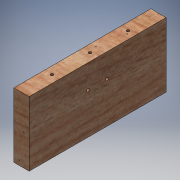
# Autodesk Inventor part: licht_200_side_left
Saved by Autodesk Inventor 2016 SP2 (Build 200236200, 236)
## iProperties
Created: 2018-01-11
Part Number: licht_200_side_left
Material: Spanplatte
Document SubType Name: Blech
Designer: schueler
Density: 1 g/cm^3
Sheet Metal Rule: Standard_mm
Appearance: Birke - natur- poliert
Mass: 154.711 g
Surface Area: 288.071 cm^2
Volume: 154.711 cm^3
Author: schueler
Autodesk Inventor part; units mm, degrees
ref_plane "YZ Plane" through (0, 0, 0) normal (1, 0, 0) x (0, 1, 0)
ref_plane "XZ Plane" through (0, 0, 0) normal (0, 1, 0) x (-1, 0, 0)
ref_plane "XY Plane" through (0, 0, 0) normal (0, 0, 1) x (1, 0, 0)
sketch "Skizze1" plane through (0, 0, 0) normal (1, 0, 0) x (0, 1, 0)
  line L0 (0, 0) -> (144, 0)
  line L1 (144, 0) -> (144, -68)
  line L2 (144, -68) -> (0, -68)
  line L3 (0, -68) -> (0, 0)
  dimension "d0" = 144
  dimension "d1" = 68
  constraints: 8 end point, 2 parallel, 1 horizontal, 1 perpendicular
  measures "d0" distance of L1.end L2.end
  measures "d1" distance of L0.end L1.end
extrude "Extrusion1" add sketch "Skizze1" along normal blind 16
sketch "Skizze2" plane through (0, 0, 0) normal (0, 0, 1) x (1, 0, 0)
  line L0 (0, 0) -> (0, 144) construction
  line L1 (0, 72) -> (16, 72) construction
  line L2 (16, 144) -> (16, 0) construction
  line L3 (0, 144) -> (16, 144) construction
  line L4 (8, 144) -> (8, 0) construction
  line L5 (0, 144) -> (16, 144) construction
  line L6 (0, 0) -> (16, 0) construction
  line L7 (0, 144) -> (16, 144) construction
  line L8 (16, 144) -> (16, 0) construction
  line L9 (16, 0) -> (0, 0) construction
  line L10 (0, 0) -> (0, 144) construction
  line L11 (0, 112) -> (16, 112) construction
  line L12 (0, 32) -> (16, 32) construction
  point P0 (8, 112)
  point P1 (8, 72)
  point P2 (8, 32)
  dimension "d4" = 40
  dimension "d5" = 40
  constraints: 16 end point, 7 midpoint, 4 point on line, 3 perpendicular, 2 parallel, 1 horizontal, 1 vertical
  measures "d4" distance of L1.end L11.end
  measures "d5" distance of L1.end L12.end
hole "Bohrung1" at (8, 112, 0) at (8, 72, 0) at (8, 32, 0) direction (0, 0, -1) diameter 3 depth 30 tip angle 118
sketch "Skizze3" plane through (0, 144, 0) normal (0, 1, 0) x (1, 0, 0)
  line L0 (0, 0) -> (16, 0)
  line L1 (16, 0) -> (16, 68)
  line L2 (16, 68) -> (0, 68)
  line L3 (0, 68) -> (0, 0)
  line L4 (8, 0) -> (8, 68) construction
  line L5 (0, 68) -> (16, 68) construction
  line L6 (16, 0) -> (16, 68) construction
  line L7 (16, 34) -> (0, 34) construction
  line L8 (0, 68) -> (0, 0) construction
  line L9 (0, 14) -> (16, 14) construction
  line L10 (0, 54) -> (16, 54) construction
  point P0 (8, 14)
  point P1 (8, 54)
  dimension "d13" = 14
  dimension "d22" = 14
  constraints: 16 end point, 6 midpoint, 4 point on line, 3 parallel, 2 perpendicular, 1 horizontal
  measures "d13" distance of L2.end L10.start
  measures "d22" distance between parallel lines of L0 L9
hole "Bohrung2" at (8, 144, -14) at (8, 144, -54) direction (0, -1, 0) diameter 3 depth 25 tip angle 118
sketch "Skizze4" plane through (0, 0, -68) normal (0, 0, -1) x (-1, 0, 0)
  line L0 (0, 0) -> (-16, 0) construction
  line L1 (-16, 0) -> (-16, 144) construction
  line L2 (-16, 144) -> (0, 144) construction
  line L3 (0, 144) -> (0, 0) construction
  line L4 (-8, 0) -> (-8, 144) construction
  line L5 (-16, 144) -> (-16, 0) construction
  line L6 (-16, 72) -> (0, 72) construction
  circle A0 centre (-8, 72) radius 1.5 construction
  point P0 (-8, 112)
  point P1 (-8, 32)
  dimension "d23" = 40
  dimension "d24" = 40
  constraints: 12 end point, 4 midpoint, 2 parallel, 2 point on line, 1 coincident, 1 horizontal, 1 perpendicular
  measures "d23" distance of point (-8, 112) point (-8, 72)
  measures "d24" distance of point (-8, 32) point (-8, 72)
hole "Bohrung3" at (8, 72, -68) at (8, 112, -68) at (8, 32, -68) direction (0, 0, 1) diameter 3 depth 30 tip angle 118
sketch "Skizze6" plane through (0, 0, 0) normal (-1, 0, 0) x (0, 0, 1)
  line L0 (0, 0) -> (-68, 0) construction
  line L1 (-68, 0) -> (-68, 144) construction
  line L2 (-68, 144) -> (0, 144) construction
  line L3 (0, 144) -> (0, 0) construction
  line L4 (0, 144) -> (0, 0) construction
  line L5 (0, 72) -> (-68, 72) construction
  line L6 (-68, 70.5) -> (-68, 73.5) construction
  line L7 (0, 0) -> (-68, 0) construction
  line L8 (-34, 0) -> (-34, 144) construction
  line L9 (0, 144) -> (-68, 144) construction
  line L10 (-25, 82) -> (-25, 62) construction
  point P0 (-25, 72)
  dimension "d41" = 25
  dimension "d42" = 10
  constraints: 14 end point, 5 midpoint, 2 parallel, 1 horizontal, 1 perpendicular, 1 point on line, 1 vertical
  measures "d41" distance between parallel lines of L3 L10
  measures "d42" distance from line of L5 L10.end
hole "Bohrung5" at (0, 82, -25) at (0, 62, -25) direction (1, 0, 0) diameter 3 end through all countersink diameter 8 countersink angle 90
equation "\"d48\" = Stärke"
equation "\"Biegeradius\" = Stärke"
equation "\"BreiteBiegungsfreistellung\" = Stärke"
equation "\"TiefeBiegungsfreistellung\" = 0.5 * Stärke"
equation "\"GrößeEckenfreistellung\" = 4 * Stärke"
equation "\"MinimalRest\" = 2 * Stärke"
equation "\"Übergangsradius\" = Biegeradius"
equation "\"JacobiRadiusGröße\" = Biegeradius"
equation "\"Abstandsgröße\" = Stärke"
equation "\"Stärke\" = 0.5"
